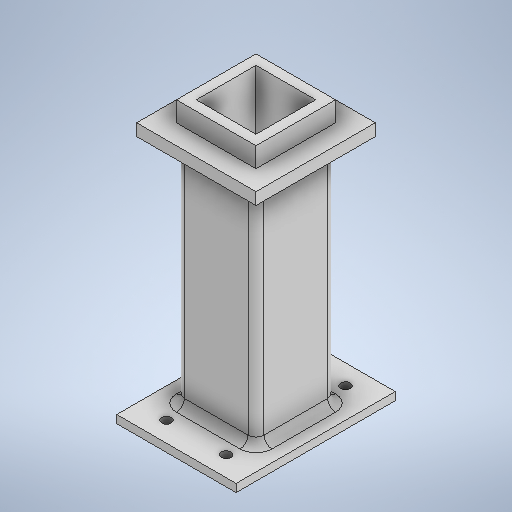
# Autodesk Inventor part: Bras caméra
Saved by Autodesk Inventor 2026.2 (Build 302298010, 298A)
## iProperties
Created: 2026-04-02
Part Number: Bras caméra
Material: Générique
Document SubType Name: Modeling
Designer: Genon
Density: 1 g/cm^3
Appearance: Par défaut
Author: Genon
Autodesk Inventor part; units mm, degrees
ref_plane "YZ Plane" through (0, 0, 0) normal (1, 0, 0) x (0, 1, 0)
ref_plane "XZ Plane" through (0, 0, 0) normal (0, 1, 0) x (-1, 0, 0)
ref_plane "XY Plane" through (0, 0, 0) normal (0, 0, 1) x (1, 0, 0)
sketch "Esquisse1" plane through (0, 0, 0) normal (0, 1, 0) x (-1, 0, 0)
  line L0 (-15, 20) -> (15, 20)
  line L1 (15, 20) -> (15, -20)
  line L2 (15, -20) -> (-15, -20)
  line L3 (-15, -20) -> (-15, 20)
  line L4 (-15, 20) -> (15, -20) construction
  line L5 (15, 20) -> (-15, -20) construction
  point P0 (0, 0)
  dimension "d0" = 30
  dimension "d1" = 40
  constraints: 12 end point, 2 midpoint, 2 parallel, 1 horizontal, 1 perpendicular
  measures "d0" distance of L1.end L2.end
  measures "d1" distance of L0.end L1.end
extrude "Extrusion1" add sketch "Esquisse1" along normal blind 2
sketch "Esquisse2" plane through (0, 2, 0) normal (0, 1, 0) x (1, 0, 0)
  line L0 (10, -10) -> (-10, -10)
  line L1 (-10, -10) -> (-10, 10)
  line L2 (-10, 10) -> (10, 10)
  line L3 (10, 10) -> (10, -10)
  line L4 (10, -10) -> (-10, 10) construction
  line L5 (-10, -10) -> (10, 10) construction
  point P0 (0, 0)
  dimension "d4" = 20
  dimension "d5" = 20
  constraints: 12 end point, 2 midpoint, 2 parallel, 1 horizontal, 1 perpendicular
  measures "d4" distance of L1.end L2.end
  measures "d5" distance of L0.end L1.end
extrude "Extrusion2" add sketch "Esquisse2" along normal blind 66
sketch "Esquisse3" plane through (0, 68, 0) normal (0, 1, 0) x (1, 0, 0)
  line L0 (7.5, 7.5) -> (-7.5, 7.5)
  line L1 (-7.5, 7.5) -> (-7.5, -7.5)
  line L2 (-7.5, -7.5) -> (7.5, -7.5)
  line L3 (7.5, -7.5) -> (7.5, 7.5)
  line L4 (7.5, 7.5) -> (-7.5, -7.5) construction
  line L5 (-7.5, 7.5) -> (7.5, -7.5) construction
  point P0 (0, 0)
  dimension "d9" = 15
  dimension "d10" = 15
  constraints: 12 end point, 2 midpoint, 2 parallel, 1 horizontal, 1 perpendicular
  measures "d9" distance of L2.end L1.end
  measures "d10" distance of L1.end L0.end
extrude "Extrusion3" cut sketch "Esquisse3" against normal through all
sketch "Esquisse4" plane through (0, 2, 0) normal (0, 1, 0) x (1, 0, 0)
  line L0 (0, 0) -> (0, -15)
  line L1 (0, -15) -> (-7.5, -15)
  line L2 (0, 0) -> (0, 15)
  line L3 (0, 15) -> (-7.5, 15)
  point P0 (7.5, -15)
  point P1 (7.5, 15)
  point P2 (7.5, 15)
  dimension "d13" = 15
  dimension "d14" = 7.5
  dimension "d15" = 15
  dimension "d16" = 7.5
  constraints: 8 end point, 3 coincident, 3 symmetric about line, 2 perpendicular, 2 vertical
  measures "d13" distance of L0.start L0.end
  measures "d14" distance of L0.end L1.end
  measures "d15" distance of L0.start L2.end
  measures "d16" distance of L2.end L3.end
hole "Perçage1" at (-7.5, 2, 15) at (7.5, 2, 15) at (-7.5, 2, -15) at (7.5, 2, -15) direction (0, -1, 0) diameter 2.459 end through all thread size "M3x0.5" class "6H" standard "ISO Metric profile"
sketch "Esquisse5" plane through (10, 2, -10) normal (0, 0, -1) x (-1, 0, 0)
  point P0 (10, -2)
sketch "Esquisse6" plane through (10, 2, -10) normal (0, 0, -1) x (-1, 0, 0)
  line L0 (0, 66) -> (20, 66) projected
  line L1 (0, 66) -> (0, 61)
  line L2 (0, 0) -> (0, 66) projected
  line L3 (20, 0) -> (20, 66) projected
  line L4 (0, 61) -> (20, 61)
  line L5 (20, 61) -> (20, 58)
  line L6 (20, 58) -> (0, 58)
  line L7 (0, 58) -> (0, 61)
  point P0 (10, -2)
  point P1 (0, 58)
  dimension "d24" = 5
  dimension "d25" = 3
  constraints: 10 end point, 2 parallel, 2 point on line, 1 horizontal, 1 perpendicular
  measures "d24" distance of L0.start L1.end
  measures "d25" distance of L4.end L5.end
extrude "Extrusion4" add sketch "Esquisse6" along normal blind 5 contours L4 L3 L6 L2
sketch "Esquisse7" plane through (-10, 2, 10) normal (0, 0, 1) x (1, 0, 0)
  line L0 (0, 66) -> (20, 66) projected
  line L1 (0, 66) -> (0, 61)
  line L2 (0, 0) -> (0, 66) projected
  line L3 (20, 0) -> (20, 58) projected
  line L4 (0, 61) -> (20, 61)
  line L5 (20, 61) -> (20, 58)
  line L6 (20, 58) -> (0, 58)
  line L7 (0, 58) -> (0, 61)
  point P0 (10, -2)
  point P1 (0, 58)
  dimension "d28" = 5
  dimension "d29" = 3
  constraints: 10 end point, 2 parallel, 2 point on line, 1 horizontal, 1 perpendicular
  measures "d28" distance of L0.start L1.end
  measures "d29" distance of L4.end L5.end
extrude "Extrusion5" add sketch "Esquisse7" along normal blind 5
sketch "Esquisse8" plane through (10, 2, 10) normal (1, 0, 0) x (0, 0, -1)
  line L0 (-5, 61) -> (-5, 58) projected
  line L1 (20, 58) -> (25, 58) projected
  line L2 (-5, 61) -> (25, 61)
  line L3 (25, 61) -> (25, 58)
  line L4 (25, 58) -> (-5, 58)
  line L5 (-5, 58) -> (-5, 61)
  point P0 (10, -2)
  constraints: 8 end point, 2 parallel, 1 horizontal, 1 perpendicular
extrude "Extrusion6" add sketch "Esquisse8" along normal blind 5
sketch "Esquisse9" plane through (-10, 2, -10) normal (-1, 0, 0) x (0, 0, 1)
  line L0 (-5, 58) -> (-5, 61) projected
  line L1 (25, 61) -> (25, 58) projected
  line L2 (-5, 61) -> (25, 61)
  line L3 (25, 61) -> (25, 58)
  line L4 (25, 58) -> (-5, 58)
  line L5 (-5, 58) -> (-5, 61)
  point P0 (10, -2)
  constraints: 8 end point, 2 parallel, 1 horizontal, 1 perpendicular
extrude "Extrusion7" add sketch "Esquisse9" along normal blind 5
fillet "Congé2" radius 2 8 edges at (10, 31, -10) (10, 31, 10) (10, 2, 0) (0, 2, -10) (-10, 31, -10) (-10, 2, 0) (-10, 31, 10) (0, 2, 10)
fillet "Congé3" radius 2 8 edges at (-9.4142, 60, -9.4142) (0, 60, -10) (9.4142, 60, -9.4142) (10, 60, 0) (9.4142, 60, 9.4142) (0, 60, 10) (-9.4142, 60, 9.4142) (-10, 60, 0)
